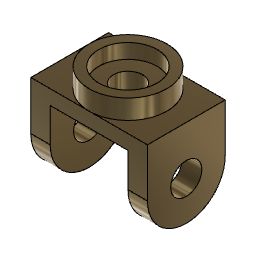
1) 3d sketch v1 (Autodesk Fusion 360 design; units mm, degrees)
Autodesk Fusion 360 part; units mm, degrees
sketch "Sketch1" plane through (0, 0, 0) normal (0, 0, 1) x (1, 0, 0)
  line L0 (60, -40) -> (-60, -40)
  line L1 (-60, -40) -> (-60, 40)
  line L2 (-60, 40) -> (60, 40)
  line L3 (60, 40) -> (60, -40)
  line L4 (60, -40) -> (-60, 40) construction
  line L5 (-60, -40) -> (60, 40) construction
  dimension "d1" = 120
  dimension "d2" = 80
  constraint horizontal L0
  constraint perpendicular L0 L1
  constraint parallel L0 L2
  constraint parallel L1 L3
  constraint coincident L4 origin
  constraint coincident L5 origin
  measures "d1" distance of L1.end L2.end
  measures "d2" distance of L0.end L1.end
extrude "Extrude1" add sketch "Sketch1" against normal blind 15
sketch "Sketch2" plane through (0, 0, 0) normal (0, 0, 1) x (-1, 0, 0)
  line L0 (-60, -40) -> (60, -40)
  line L1 (60, -40) -> (60, 40)
  line L2 (60, 40) -> (-60, 40)
  line L3 (-60, 40) -> (-60, -40)
  circle A0 centre (0, 0) radius 40
  dimension "d5" = 80
  constraint coincident A0.centre origin
  measures "d5" diameter of A0
extrude "Extrude2" add sketch "Sketch2" along normal blind 20 contours A0
sketch "Sketch3" plane through (0, 0, 20) normal (0, 0, 1) x (-1, 0, 0)
  circle A0 centre (0, 0) radius 40
  circle A1 centre (0, 0) radius 30
  dimension "d8" = 60
  constraint concentric A0 A1
  measures "d8" diameter of A1
extrude "Extrude3" cut sketch "Sketch3" against normal blind 15 contours A1
sketch "Sketch4" plane through (0, 0, 5) normal (0, 0, 1) x (-1, 0, 0)
  circle A0 centre (0, 0) radius 30
  circle A1 centre (0, 0) radius 15
  dimension "d11" = 30
  constraint concentric A0 A1
  measures "d11" diameter of A1
extrude "Extrude4" cut sketch "Sketch4" against normal blind 20 contours A1
sketch "Sketch5" plane through (60, 0, 0) normal (1, 0, 0) x (0, 1, 0)
  line L0 (40, 0) -> (-40, 0)
  line L1 (-40, 0) -> (-40, -15)
  line L2 (-40, -15) -> (40, -15)
  line L3 (40, -15) -> (40, 0)
  line L4 (-40, -15) -> (40, -15)
  line L5 (40, -15) -> (40, -50)
  line L6 (40, -50) -> (-40, -50)
  line L7 (-40, -50) -> (-40, -15)
  arc A0 (-40, -50) -> (40, -50) centre (0, -50) ccw
  circle A1 centre (0, -50) radius 16
  dimension "d14" = 35
  dimension "d15" = 32
  constraint horizontal L4
  constraint vertical L5
  constraint horizontal L6
  constraint vertical L7
  constraint coincident L1.end L2.start
  constraint midpoint L6 A0.centre
  constraint concentric A0 A1
  measures "d14" distance of L1.end L6.end
  measures "d15" diameter of A1
extrude "Extrude5" add sketch "Sketch5" against normal blind 20 contours L2 L4 L5 L6 L7 A1 | L6 A0 A1
mirror "Mirror1" about plane through (0, 0, 0) normal (1, 0, 0) of "Extrude5"
